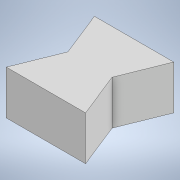
# Autodesk Inventor part: dishConnector
Saved by Autodesk Inventor 2022.1 (Build 261234020, 234B)
## iProperties
Created: 2021-10-10
Part Number: dishConnector
Material: Generic
Document SubType Name: Modeling
Designer: yiunf
Density: 1 g/cm^3
Appearance: Default
Author: yiunf
## iProperties of the stored document dishConnector_3DPrint.ipt
Created: 2021-10-10
Part Number: dishConnector_3DPrint
Material: Generic
Document SubType Name: Modeling
Designer: yiunf
Density: 1 g/cm^3
Appearance: Default
Author: yiunf
Autodesk Inventor part; units mm, degrees
ref_plane "YZ Plane" through (0, 0, 0) normal (1, 0, 0) x (0, 1, 0)
ref_plane "XZ Plane" through (0, 0, 0) normal (0, 1, 0) x (-1, 0, 0)
ref_plane "XY Plane" through (0, 0, 0) normal (0, 0, 1) x (1, 0, 0)
sketch "Sketch1" plane through (0, 0, 0) normal (0, 1, 0) x (-1, 0, 0)
  line L0 (0, 0) -> (10, 0)
  line L1 (5, 0) -> (5, -10)
  line L2 (10, -10) -> (0, -10)
  line L3 (5, -5) -> (7.5, -5)
  line L4 (7.5, -5) -> (10, 0)
  line L5 (7.5, -5) -> (10, -10)
  line L6 (5, -5) -> (2.5, -5)
  line L7 (2.5, -5) -> (0, -10)
  line L8 (2.5, -5) -> (0, 0)
  line L9 (5, 0) -> (9.5, 0)
  line L10 (9.5, 0) -> (7.5, -5)
  line L11 (5, 0) -> (0.5, 0)
  line L12 (0.5, 0) -> (2.5, -5)
  line L13 (2.5, -5) -> (0.5, -10)
  line L14 (7.5, -5) -> (9.5, -10)
  dimension "d0" = 10
  dimension "d1" = 10
  dimension "d2" = 2.5
  dimension "d3" = 2.5
  dimension "d4" = 4.5
  dimension "d5" = 4.5
  constraints: 30 end point, 5 point on line, 4 parallel, 3 horizontal, 2 midpoint, 1 vertical
  measures "d0" distance of L0.start L0.end
  measures "d1" distance of L1.start L1.end
  measures "d2" distance of L3.start L3.end
  measures "d3" distance of L3.start L6.end
  measures "d4" distance of L1.start L9.end
  measures "d5" distance of L1.start L11.end
extrude "Extrusion1" add sketch "Sketch1" along normal blind 5 contours L0 L1 L6 L12 | L6 L1 L2 L13 | L0 L10 L3 L1 | L3 L14 L2 L1
body "Solid1"
